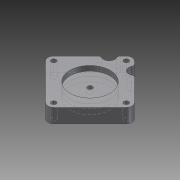
# Autodesk Inventor part: MatingPlates
Saved by Autodesk Inventor 2011 SP2 (Build 150309200, 309)
## iProperties
Created: 2014-05-12
Part Number: MatingPlates
Document SubType Name: Modeling
Designer: Maurice Woods
Density: 1 g/cm^3
Author: Maurice Woods
Autodesk Inventor part; units mm, degrees
ref_plane "YZ Plane" through (0, 0, 0) normal (1, 0, 0) x (0, 1, 0)
ref_plane "XZ Plane" through (0, 0, 0) normal (0, 1, 0) x (-1, 0, 0)
ref_plane "XY Plane" through (0, 0, 0) normal (0, 0, 1) x (1, 0, 0)
sketch "Sketch1" plane through (0, 0, 0) normal (0, 0, 1) x (1, 0, 0)
  line L0 (0, 25.4) -> (-25.4, 0) construction
  line L1 (-25.4, 0) -> (0, -25.4) construction
  line L2 (0, -25.4) -> (25.4, 0) construction
  line L3 (25.4, 0) -> (0, 25.4) construction
  line L4 (0, 25.4) -> (0, -25.4) construction
  line L5 (-25.4, 0) -> (25.4, 0) construction
  line L6 (-28.2284, 2.8284) -> (-2.8284, 28.2284)
  line L7 (2.8284, 28.2284) -> (28.2284, 2.8284)
  line L8 (28.2284, -2.8284) -> (2.8284, -28.2284)
  line L9 (-2.8284, -28.2284) -> (-28.2284, -2.8284)
  arc A0 (2.8284, 28.2284) -> (-2.8284, 28.2284) centre (0, 25.4) ccw
  arc A1 (28.2284, -2.8284) -> (28.2284, 2.8284) centre (25.4, 0) ccw
  arc A2 (-2.8284, -28.2284) -> (2.8284, -28.2284) centre (0, -25.4) ccw
  arc A3 (-28.2284, 2.8284) -> (-28.2284, -2.8284) centre (-25.4, 0) ccw
  circle A4 centre (0, 0) radius 10.0263 construction
  circle A5 centre (0, 0) radius 14.0263
  dimension "d0" = 4
  dimension "d1" = 4
  dimension "d2" = 25.4
  dimension "d22" = 20.0526
  dimension "d23" = 4
  constraints: 20 end point, 8 point on circle, 8 tangent, 6 centre point, 4 parallel, 3 equal radius, 3 perpendicular, 2 coincident, 1 midpoint, 1 vertical, 3 other
  measures "d0" distance between parallel lines of L8 L2
  measures "d1" radius of A0
  measures "d2" distance of point (0, 0) L0.end
  measures "d22" diameter of A4
  measures "d23" radial gap between concentric circles of A5 A4
extrude "Extrusion1" add sketch "Sketch1" along normal mid plane 10
extrude "Extrusion2" add sketch "Sketch1" along normal mid plane 3 contours A5
sketch "Sketch2" plane through (0, 0, 5) normal (0, 0, 1) x (1, 0, 0)
  arc A0 (28.2284, -2.8284) -> (28.2284, 2.8284) centre (25.4, 0) ccw projected
  arc A1 (2.8284, 28.2284) -> (-2.8284, 28.2284) centre (0, 25.4) ccw projected
  arc A2 (-28.2284, 2.8284) -> (-28.2284, -2.8284) centre (-25.4, 0) ccw projected
  arc A3 (-2.8284, -28.2284) -> (2.8284, -28.2284) centre (0, -25.4) ccw projected
  point P0 (0, 0)
hole "Hole1" at (0, 25.4, 5) at (-25.4, 0, 5) at (0, -25.4, 5) at (25.4, 0, 5) at (0, 0, 5) direction (0, 0, -1) diameter 3.4 end through all clearance for "Socket Head Cap Screw" size "M3" standard "Ansi Metric M Profile"
sketch "Sketch3" plane through (0, 0, -5) normal (0, 0, -1) x (-1, 0, 0)
  circle A0 centre (0, 0) radius 14.0263 construction
  arc A1 (2.8284, 28.2284) -> (-2.8284, 28.2284) centre (0, 25.4) ccw construction
  line L0 (-28.2284, 2.8284) -> (-2.8284, 28.2284) construction
  circle A2 centre (-8.8388, 22.218) radius 4
  line L1 (0, 0) -> (0, 25.4) construction
  circle A3 centre (8.8388, 22.218) radius 4
  dimension "d26" = 8.5
  dimension "d27" = 8
  constraints: 2 centre point, 2 end point, 1 point on line, 1 symmetric about line, 1 other
  measures "d26" distance of L0.end A2.centre
  measures "d27" diameter of A2
extrude "Extrusion3" cut sketch "Sketch3" against normal through all
fillet "Fillet1" radius 2 4 edges at (6.0104, 25.0464, 0) (11.6673, 19.3896, 0) (-6.0104, 25.0464, 0) (-11.6673, 19.3896, 0)
equation "\"d2\" = LengthA"
equation "\"d22\" = 2 * LengthM"
equation "\"LengthM\" = 10.02632"
equation "\"LengthA\" = 25.4"
body "Solid1"
